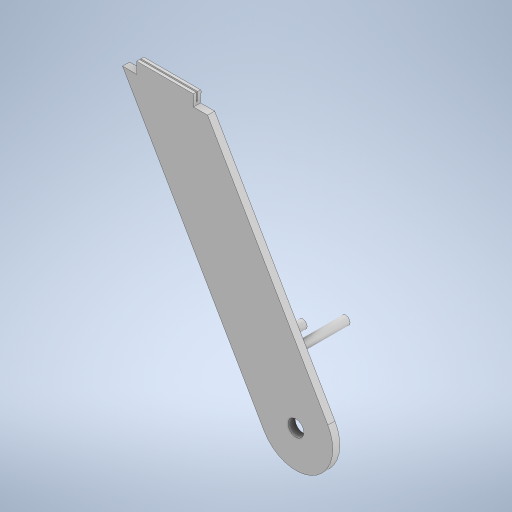
# Autodesk Inventor part: bacak
Saved by Autodesk Inventor 2023.2 (Build 272271000, 271)
## iProperties
Created: 2022-11-26
Part Number: bacak
Material: Generic
Document SubType Name: Modeling
Designer: omrfrkmll
Density: 1 g/cm^3
Appearance: Default
Author: omrfrkmll
Autodesk Inventor part; units mm, degrees
ref_plane "YZ Plane" through (0, 0, 0) normal (1, 0, 0) x (0, 1, 0)
ref_plane "XZ Plane" through (0, 0, 0) normal (0, 1, 0) x (-1, 0, 0)
ref_plane "XY Plane" through (0, 0, 0) normal (0, 0, 1) x (1, 0, 0)
sketch "Sketch1" plane through (0, 0, 0) normal (0, 0, 1) x (1, 0, 0)
  line L0 (-16.8629, 0) -> (19.5362, 0)
  line L1 (0, 12.2153) -> (0, -13.8193)
  line L2 (-10, 1.5) -> (10, 1.5)
  line L3 (10, 1.5) -> (10, -1.5)
  line L4 (10, -1.5) -> (-10, -1.5)
  line L5 (-10, -1.5) -> (-10, 1.5)
  point P0 (0, 0)
  point P1 (0, -1.5)
  point P2 (0, 1.5)
  dimension "d0" = 3
  dimension "d1" = 20
  constraints: 12 end point, 3 horizontal, 2 parallel, 2 vertical, 1 perpendicular, 3 other
  measures "d0" distance between parallel lines of L4 L2
  measures "d1" distance between parallel lines of L5 L3
sketch "Sketch3" plane through (0, 0, 0) normal (0, 0, 1) x (1, 0, 0)
  line L0 (0, 4.1951) -> (0, -4.771)
  line L1 (15, -1.5) -> (57.438, -75.0048)
  line L2 (-15, -1.5) -> (34.938, -87.9952)
  line L3 (0, -1.5) -> (34.9904, -62.1052)
  arc A0 (34.938, -87.9952) -> (57.438, -75.0048) centre (46.188, -81.5) ccw
  line L4 (-17.5915, 0) -> (22.0991, 0)
  line L5 (-15, -1.5) -> (15, -1.5)
  point P0 (0, -0.2879)
  dimension "d20" = 30
  dimension "d36" = 3
  dimension "d37" = 80
  dimension "d38" = 12.9904
  dimension "d39" = 124.2104
  dimension "d40" = 44.1981
  dimension "d41" = 8.3903
  dimension "d42" = 0.5758
  dimension "d43" = 3
  dimension "d44" = 35.1831
  constraints: 12 end point, 3 horizontal, 2 parallel, 2 point on circle, 2 tangent, 2 vertical, 1 centre point, 1 midpoint, 1 point on line, 1 symmetric about line
  measures "d20" distance of L2.start L1.start
  measures "d36" diameter of L5 L4
  measures "d37" distance from line of A0.centre L5
  measures "d38" radius of A0
  measures "d39" diameter of L3.end L4
  measures "d40" diameter of L4.end L0
  measures "d41" diameter of L0.start L4
  measures "d42" diameter of point (0, -0.288) L4
  measures "d43" diameter of L3.start L4
  measures "d44" diameter of L4.start L0
extrude "Extrusion1" add sketch "Sketch3" along normal mid plane 2.5
sketch "Sketch5" plane through (0, 0, 1.25) normal (0, 0, 1) x (1, 0, 0)
  arc A0 (34.938, -87.9952) -> (57.438, -75.0048) centre (46.188, -81.5) ccw projected
  point P0 (0, 0)
  point P1 (38.391, -42.0144)
  constraints: 1 coincident
hole "Hole1" at (46.188, -81.5, 1.25) direction (0, 0, -1) diameter 5.6 end through all
sketch "Sketch6" plane through (0, 0, 1.25) normal (0, 0, 1) x (1, 0, 0)
  line L0 (21.1799, -20.6847) -> (35.9337, -46.239)
  line L1 (4.4808, -26.761) -> (20.9112, -55.2193)
  line L2 (57.438, -75.0048) -> (15, -1.5) projected
  line L3 (28.5854, -68.5113) -> (43.7408, -59.7613)
  circle A0 centre (43.7408, -59.7613) radius 1.55
  circle A1 centre (28.5854, -68.5113) radius 1.55
  circle A2 centre (46.188, -81.5) radius 2.8 projected
  line L4 (46.188, -81.5) -> (10.4204, -19.5487)
  line L5 (43.7408, -59.7613) -> (46.188, -81.5)
  point P0 (0, 0)
  point P1 (38.391, -42.0144)
  dimension "d25" = 17.5
  dimension "d26" = 3.1
  dimension "d27" = 3.1
  dimension "d32" = 21.876
  constraints: 10 end point, 2 centre point, 2 coincident, 2 parallel, 2 point on line, 1 perpendicular, 2 other
  measures "d25" distance between parallel lines of L1 L0
  measures "d26" diameter of A0
  measures "d27" diameter of A1
  measures "d32" distance of L4.start L5.start
extrude "Extrusion3" add sketch "Sketch6" against normal blind 20 contours A1 | A0 L5 L3 | L3 L5 A0
extrude "Extrusion4" add sketch "Sketch1" along normal mid plane 2.5
sketch "Sketch7" plane through (10, -1.5, 1.25) normal (1, 0, 0) x (0, 0, -1)
  line L0 (0, 0) -> (0, 3) projected
  line L1 (0, 3) -> (2.5, 3)
  line L2 (2.5, 3) -> (2.5, 4)
  line L3 (2.5, 4) -> (0, 4)
  line L4 (0, 4) -> (0, 3)
  line L5 (2.5, 4) -> (3, 3)
  line L6 (3, 3) -> (2.5, 3)
  point P0 (1.25, 1.5)
  dimension "d45" = 1
  dimension "d46" = 0.5
  constraints: 12 end point, 2 horizontal, 2 parallel, 1 perpendicular
  measures "d45" distance between parallel lines of L1 L3
  measures "d46" distance from line of L2 L5.end
extrude "Extrusion5" add sketch "Sketch7" against normal up to surface (20 mm away)
sketch "Sketch8" plane through (10, -1.5, 1.25) normal (1, 0, 0) x (0, 0, -1)
  line L0 (2.5, 4) -> (0, 4) projected
  line L1 (1.25, 4) -> (1.25, -0.4591)
  line L2 (1, 4.1974) -> (1.5, 4.1974)
  line L3 (1.5, 4.1974) -> (1.5, 1)
  line L4 (1.5, 1) -> (1, 1)
  line L5 (1, 1) -> (1, 4.1974)
  line L6 (2.5, 0) -> (0, 0) projected
  point P0 (1.25, 1.5)
  dimension "d49" = 1
  dimension "d50" = 0.5
  constraints: 10 end point, 2 parallel, 1 horizontal, 1 midpoint, 1 perpendicular, 1 vertical, 1 other
  measures "d49" distance between parallel lines of L6 L4
  measures "d50" distance between parallel lines of L5 L3
extrude "Extrusion6" cut sketch "Sketch8" against normal up to surface (20 mm away)
body "Solid1"
